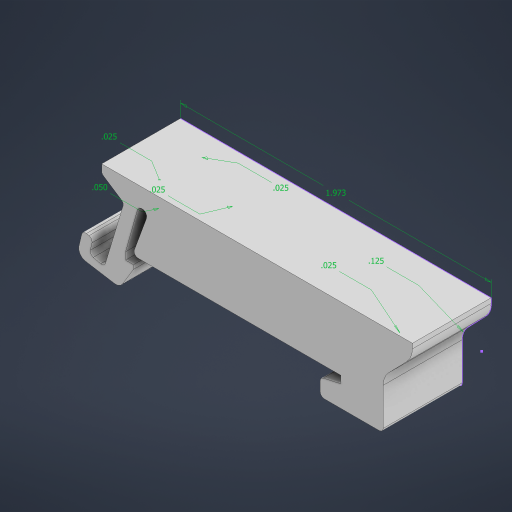
# Autodesk Inventor part: Din Mount Revised
Saved by Autodesk Inventor 2024 (Build 280153000, 153)
## iProperties
Created: 2025-02-15
Part Number: Din Mount Revised
Material: Generic
Document SubType Name: Modeling
Designer: Tommy Rohmann
Density: 1 g/cm^3
Appearance: Default
Author: Tommy Rohmann
Autodesk Inventor part; units mm, degrees
ref_plane "YZ Plane" through (0, 0, 0) normal (1, 0, 0) x (0, 1, 0)
ref_plane "XZ Plane" through (0, 0, 0) normal (0, 1, 0) x (-1, 0, 0)
ref_plane "XY Plane" through (0, 0, 0) normal (0, 0, 1) x (1, 0, 0)
sketch "Sketch1" plane through (0, 0, 0) normal (0, 0, 1) x (1, 0, 0)
  line L0 (-23.7457, -2.6209) -> (-23.4724, -1.4509)
  line L1 (-24.3668, -0.5899) -> (-23.9463, -0.6881)
  line L2 (-25.1296, -1.0638) -> (-25.5805, -2.994)
  line L3 (-23.2718, -3.3837) -> (-22.0616, -3.6664)
  line L4 (-21.3092, -3.2312) -> (-19.5512, 2.6025)
  line L5 (-16.7854, -1.1616) -> (-18.0554, -1.1616)
  line L6 (-16.7854, 0.5921) -> (-16.9615, 0.1084)
  line L7 (-18.464, 6.2104) -> (-21.371, -3.4363)
  line L8 (23.4824, -3.8755) -> (23.4824, 2.1323)
  line L9 (13.9562, -4.5105) -> (22.8474, -4.5105)
  line L10 (13.3212, -2.3102) -> (13.3212, -3.8755)
  line L11 (16.6232, -1.0769) -> (13.8205, -1.6899)
  line L12 (16.6232, 0.1084) -> (16.6232, -1.0769)
  line L13 (-16.0547, 0.1084) -> (16.6232, 0.1084)
  arc A0 (-18.0554, 0.0145) -> (-18.0554, -1.1616) centre (-4.9838, -0.5736) ccw
  arc A1 (-16.5514, 5.5422) -> (-16.5517, 5.5414) centre (-15.8594, 5.29) ccw
  line L14 (-16.6515, 0.9604) -> (-14.6821, 6.3764)
  line L15 (-18.0554, 0.0145) -> (-16.145, 6.8172)
  line L16 (-16.7854, -1.8088) -> (-18.5413, -4.7223)
  line L17 (-19.8373, -5.3195) -> (-24.5521, -4.5357)
  line L18 (-16.7854, -1.1616) -> (-16.7854, -1.8088)
  arc A2 (-25.5805, -2.994) -> (-24.5521, -4.5357) centre (-24.3438, -3.2829) ccw
  arc A3 (-19.8373, -5.3195) -> (-18.5413, -4.7223) centre (-19.629, -4.0667) ccw
  arc A4 (-24.3668, -0.5899) -> (-25.1296, -1.0638) centre (-24.5112, -1.2082) ccw
  arc A5 (-23.4724, -1.4509) -> (-23.9463, -0.6881) centre (-24.0908, -1.3064) ccw
  arc A6 (-23.7457, -2.6209) -> (-23.2718, -3.3837) centre (-23.1274, -2.7653) ccw
  arc A7 (-22.0616, -3.6664) -> (-21.3092, -3.2312) centre (-21.9172, -3.048) ccw
  arc A8 (13.8205, -1.6899) -> (13.3212, -2.3102) centre (13.9562, -2.3102) ccw
  arc A9 (13.3212, -3.8755) -> (13.9562, -4.5105) centre (13.9562, -3.8755) ccw
  arc A10 (22.8474, -4.5105) -> (23.4824, -3.8755) centre (22.8474, -3.8755) ccw
  arc A11 (-14.7114, 6.296) -> (-16.1528, 6.7894) centre (-15.4136, 6.5968) ccw
  line L19 (-24.7257, -0.6105) -> (-20.0096, 1.0815)
  line L20 (-21.9172, 10.3524) -> (28.1843, 10.3524)
  line L21 (28.1843, 10.3524) -> (28.1843, 9.5643)
  line L22 (27.2923, 7.3579) -> (24.3744, 4.3388)
  arc A12 (24.3744, 4.3388) -> (23.4824, 2.1323) centre (26.6574, 2.1323) ccw
  arc A13 (27.2923, 7.3579) -> (28.1843, 9.5643) centre (25.0093, 9.5643) ccw
  line L23 (-13.5838, 2.8516) -> (-12.2444, 6.6018)
  line L24 (-11.6464, 7.0233) -> (21.1508, 7.0233)
  line L25 (21.605, 5.9445) -> (19.7384, 4.0337)
  line L26 (19.5576, 3.59) -> (19.5576, 2.638)
  line L27 (18.9226, 2.003) -> (-12.9858, 2.003)
  arc A14 (-13.5838, 2.8516) -> (-12.9858, 2.003) centre (-12.9858, 2.638) ccw
  arc A15 (-11.6464, 7.0233) -> (-12.2444, 6.6018) centre (-11.6464, 6.3883) ccw
  arc A16 (21.605, 5.9445) -> (21.1508, 7.0233) centre (21.1508, 6.3883) ccw
  arc A17 (19.7384, 4.0337) -> (19.5576, 3.59) centre (20.1926, 3.59) ccw
  arc A18 (18.9226, 2.003) -> (19.5576, 2.638) centre (18.9226, 2.638) ccw
  arc A19 (-16.6515, 0.9604) -> (-16.0547, 0.1084) centre (-16.0547, 0.7434) ccw
  line L28 (-21.6291, 8.8193) -> (-18.7251, 6.9255)
  line L29 (-21.9172, 9.3512) -> (-21.9172, 10.3524)
  arc A20 (-18.464, 6.2104) -> (-18.7251, 6.9255) centre (-19.072, 6.3936) ccw
  arc A21 (-21.9172, 9.3512) -> (-21.6291, 8.8193) centre (-21.2822, 9.3512) ccw
  point P0 (0, 0)
  point P1 (-20.0096, 1.0815)
  dimension "d1" = 1.27
  dimension "d2" = 0.635
  dimension "d3" = 0.635
  dimension "d5" = 50.1015
  dimension "d6" = 3.175
  dimension "d7" = 0.635
  dimension "d8" = 0.635
  constraints: 60 end point, 46 point on circle, 37 tangent, 22 centre point, 13 equal radius, 6 point on line, 3 perpendicular, 3 vertical, 2 horizontal
  measures "d1" radius of A2
  measures "d2" radius of A4
  measures "d3" radius of A8
  measures "d5" distance of L20.start L20.end
  measures "d6" radius of A12
  measures "d7" radius of A14
  measures "d8" radius of A20
extrude "Extrusion1" add sketch "Sketch1" along normal blind 12.7 contours A6 L3 A7 L4 L7 A20 L28 A21 L29 L20 L21 A13 L22 A12 L8 A10 L9 A9 L10 A8 L11 L12 L13 A19 L14 A11 L15 A1 A0 L5 L18 L16 A3 L17 A2 L2 A4 L1 A5 L0 | A1 L15 | L23 A15 L24 A16 L25 A17 L26 A18 L27 A14 picked at (-16.5274, 5.5086)
extrude "Extrusion2" add sketch "Sketch1" along normal blind 3.175 contours L0 A5 L1 A4 L19 L4 A7 L3 A6
body "Solid1"
